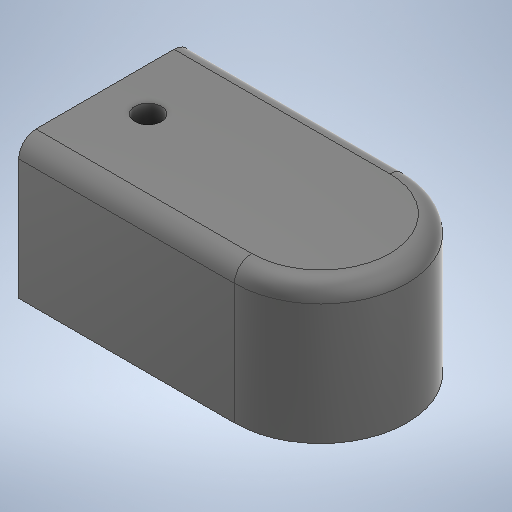
# Autodesk Inventor part: T-Frame Left Cover
Saved by Autodesk Inventor 2026.2 (Build 302298010, 298A)
## iProperties
Created: 2026-05-29
Part Number: T-Frame Left Cover
Material: ABS Plastic
Document SubType Name: Modeling
Designer: chanh
Density: 1.06 g/cm^3
Appearance: Smooth - White
Author: chanh
Autodesk Inventor part; units mm, degrees
ref_plane "YZ Plane" through (0, 0, 0) normal (1, 0, 0) x (0, 1, 0)
ref_plane "XZ Plane" through (0, 0, 0) normal (0, 1, 0) x (-1, 0, 0)
ref_plane "XY Plane" through (0, 0, 0) normal (0, 0, 1) x (1, 0, 0)
sketch "Sketch1" plane through (0, 0, 0) normal (0, 1, 0) x (-1, 0, 0)
  line L0 (5, -10) -> (-20, -10)
  line L1 (-20, -10) -> (-20, 10)
  line L2 (-20, 10) -> (5, 10)
  line L3 (5, 10) -> (5, -10)
  line L4 (5, -10) -> (-20, 10) construction
  line L5 (-20, -10) -> (5, 10) construction
  circle A0 centre (-20, 0) radius 10
  point P0 (0, 0)
  point P1 (-7.5, 0)
  point P2 (-20, 10)
  dimension "d0" = 20
  dimension "d1" = 20
  dimension "d2" = 5
  constraints: 12 end point, 3 midpoint, 2 parallel, 1 horizontal, 1 horizontal alignment, 1 perpendicular, 3 other
  measures "d0" distance from line of L1 point (0, 0)
  measures "d1" distance between parallel lines of L2 L0
  measures "d2" distance from line of L3 point (0, 0)
extrude "Extrusion1" add sketch "Sketch1" along normal mid plane 16
sketch "Sketch2" plane through (0, 8, 0) normal (0, 1, 0) x (1, 0, 0)
  point P0 (0, 0)
  point P1 (0, 0)
  constraints: 1 coincident
hole "Hole1" at (0, 8, 0) direction (0, -1, 0) diameter 3.1 end through all
sketch "Sketch3" plane through (-5, -8, 10) normal (-1, 0, 0) x (0, 0, 1)
  line L0 (-17.56, 2.94) -> (-2.44, 2.94)
  line L1 (-2.44, 2.94) -> (-2.44, 13.06)
  line L2 (-2.44, 13.06) -> (-17.56, 13.06)
  line L3 (-17.56, 13.06) -> (-17.56, 2.94)
  line L4 (-17.56, 2.94) -> (-2.44, 13.06) construction
  line L5 (-2.44, 2.94) -> (-17.56, 13.06) construction
  point P0 (-10, 8)
  dimension "d12" = 15.12
  dimension "d13" = 10.12
  constraints: 12 end point, 2 midpoint, 2 parallel, 1 horizontal, 1 perpendicular
  measures "d12" distance of L2.end L1.end
  measures "d13" distance of L0.end L1.end
extrude "Extrusion2" cut sketch "Sketch3" against normal blind 24.5
fillet "Fillet1" radius 2 3 edges at (30, 8, 0) (7.5, 8, -10) (7.5, 8, 10)
body "Solid1"
